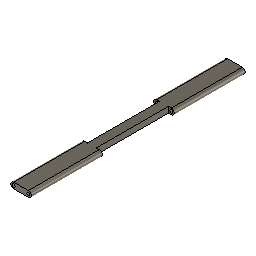
Mothbox_pro_TargetLid_asembly (Autodesk Fusion 360 archive; units mm, degrees)
design "mothbox lid hinge"
Autodesk Fusion 360 part; units mm, degrees
sketch "Sketch1" plane through (0, 0, 0) normal (0, 1, 0) x (1, 0, 0)
  line L0 (0, 0) -> (10, 0)
  line L1 (10, 0) -> (10, -4)
  line L2 (10, -4) -> (0, -4)
  line L3 (0, -4) -> (0, 0)
  circle A0 centre (0, -2) radius 2
  circle A1 centre (10, -2) radius 2
  circle A2 centre (0, -2) radius 1
  circle A3 centre (10, -2) radius 1
  dimension "d1" = 10
  dimension "d2" = 4
  dimension "d5" = 2
  dimension "d6" = 2
  constraint horizontal L0
  constraint vertical L1
  constraint horizontal L2
  constraint vertical L3
  constraint coincident L0.start L3.end
  constraint midpoint L3 A0.centre
  constraint coincident L0.start A0
  constraint midpoint L1 A1.centre
  constraint coincident L0.end A1
  constraint concentric A0 A2
  constraint concentric A1 A3
  measures "d1" distance of L0.start L0.end
  measures "d2" distance of L0.start L2.end
  measures "d5" diameter of A2
  measures "d6" diameter of A3
extrude "Extrude1" add sketch "Sketch1" along normal blind 250 contours L3 A0 A2 | L0 L2 A0 A1 | L3 A0 A2 | L1 A1 A3 | L1 A1 A3
ref_plane "WorkPlane1" through (0, 51.2, 0) normal (0, 1, 0) x (0, 0, 1)
sketch "Sketch3" plane through (0, 51.2, 0) normal (0, 1, 0) x (1, 0, 0)
  line L0 (8, -4) -> (8, 0)
  line L1 (10, -4) -> (0, -4)
  line L2 (0, 0) -> (10, 0)
  line L3 (8, -4) -> (10, -4)
  line L4 (8, 0) -> (10, 0)
  circle A0 centre (10, -2) radius 1
  circle A1 centre (10, -2) radius 1
  circle A2 centre (10, -2) radius 2
  arc A3 (10, -4) -> (10, 0) centre (10, -2) ccw
  line L5 (5, 0) -> (5, -4)
  circle A4 centre (0, -2) radius 2
  circle A5 centre (0, -2) radius 1
  line L6 (2, -4) -> (0, -4)
  line L7 (2, -4) -> (2, 0)
  line L8 (2, 0) -> (0, 0)
  dimension "d15" = 2
  constraint vertical L0
  constraint coincident L0.start L1
  constraint coincident L0.end L2
  constraint coincident L1.start L3.end
  constraint coincident L2.end L4.end
  constraint equal A0 A1
  constraint concentric A0 A2
  constraint concentric A2 A3
  constraint equal A2 A3
  constraint midpoint L2 L5.start
  constraint midpoint L1 L5.end
  constraint symmetric L0.start L5 L6.start
  constraint symmetric L0.end L5 L7.end
  constraint symmetric L1.start L5 L1.end
  constraint symmetric L2.end L5 L2.start
  constraint symmetric A0 L5 A5
  constraint symmetric A2 L5 A4
  measures "d15" distance of L0.end L2.end
extrude "Extrude3" cut sketch "Sketch3" against normal blind 49.2 contours L0 L1 L3 A2 | L0 L2 L4 A2 | A2 A3 | L1 A4 L6 L7 | A4 | L2 A4 L7 L8
ref_plane "WorkPlane2" through (0, 125, 0) normal (0, 1, 0) x (0, 0, 1)
mirror "Mirror1" about plane through (0, 125, 0) normal (0, 1, 0) of "Extrude3"
sketch "Sketch4" plane through (0, 125, 0) normal (0, 1, 0) x (1, 0, 0)
  circle A0 centre (10, -2) radius 1
  circle A1 centre (10, -2) radius 2
  circle A2 centre (0, -2) radius 1
  circle A3 centre (0, -2) radius 2
  circle A4 centre (10, -2) radius 1
  arc A5 (10, -4) -> (10, 0) centre (10, -2) ccw
  arc A6 (0, 0) -> (0, -4) centre (0, -2) ccw
  circle A7 centre (0, -2) radius 1
  line L0 (10, -4) -> (0, -4)
  line L1 (0, 0) -> (10, 0)
  line L2 (5, -4) -> (5, 0)
  line L3 (10, 0) -> (8, 0)
  line L4 (8, 0) -> (8, -4)
  line L5 (2, 0) -> (2, -4)
  dimension "d41" = 2
  constraint concentric A0 A1
  constraint concentric A2 A3
  constraint concentric A0 A4
  constraint equal A1 A5
  constraint equal A0 A4
  constraint equal A3 A6
  constraint equal A2 A7
  constraint coincident A5.start L0.start
  constraint coincident A6.end L0.end
  constraint coincident A6.start L1.start
  constraint coincident A5.end L1.end
  constraint midpoint L0 L2.start
  constraint midpoint L1 L2.end
  constraint tangent A5 L3
  constraint coincident L0 L4.end
  constraint perpendicular L0 L4
  constraint symmetric L2 L3.end L5.start
  constraint symmetric L2 L4.end L5.end
  measures "d41" distance of A5.end L3.end
extrude "Extrude8" cut sketch "Sketch4" along normal blind 24.6 and the other way blind 24.6 contours A1 A5 | A1 L1 L3 L4 | A1 L0 L4 | A3 L1 L5 | A3 L0 L5 | A3 A6
extrude "Extrude5" cut 1 faces at (3.6087, 0, 0.4789) along direction (0, 1, 0) blind 52
extrude "Extrude6" cut 1 faces at (3.6087, 250, 0.4789) along direction (0, -1, 0) blind 52
fillet "Fillet2" [rolled back] radius 1
equation "d7 = 2 mm + 49.2 mm"
